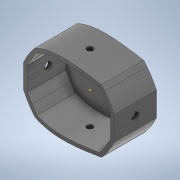
# Autodesk Inventor part: CameraHolder2
Saved by Autodesk Inventor 2021.1 (Build 251245010, 245A)
## iProperties
Created: 2023-07-02
Part Number: CameraHolder2
Material: ABS Plastic
Document SubType Name: Modeling
Designer: Drake
Density: 1.06 g/cm^3
Appearance: Smooth - White
Author: Drake
Autodesk Inventor part; units mm, degrees
ref_plane "XY Plane" through (0, 0, 0) normal (0, 0, 1) x (1, 0, 0)
sketch "Sketch1" plane through (0, 0, 0) normal (0, 0, 1) x (1, 0, 0)
  circle A0 centre (0, 0) radius 75
  line L0 (-56.086285, 49.792857) -> (-26.079044, 63.659157) construction
  line L1 (-26.079044, 63.659157) -> (7.211359, 60.092328) construction
  line L2 (7.211359, 60.092328) -> (53.805209, 52.249397) construction
  spline S0 degree 3 poles (-56.086285, 49.792857) (-26.079044, 63.659157) (7.211359, 60.092328) (53.805209, 52.249397) knots 1 1 1 1 2 2 2 2
  line L3 (-75, 0) -> (75, 0)
  line L4 (-56.086285, -49.792857) -> (-26.079044, -63.659157) construction
  line L5 (-26.079044, -63.659157) -> (7.211359, -60.092328) construction
  line L6 (7.211359, -60.092328) -> (53.805209, -52.249397) construction
  spline S1 degree 3 poles (-56.086285, -49.792857) (-26.079044, -63.659157) (7.211359, -60.092328) (53.805209, -52.249397) knots 1 1 1 1 2 2 2 2
  line L7 (0, 0) -> (0, 49.151954)
  line L8 (-75, 0) -> (-75, 20)
  line L9 (-75, 20) -> (-75, -20)
  line L10 (0, 49.151954) -> (0, -37.368697)
  line L11 (75, 20) -> (75, -20)
  arc A1 (-56.086285, 49.792857) -> (-75, 20) centre (35.126867, -29.012979) ccw
  line L12 (0, 49.151954) -> (0, 75)
  line L13 (0, 75) -> (0, -75.710243)
  line L14 (-75, 0) -> (75, 0)
  arc A2 (75, 20) -> (56.086285, 49.792857) centre (-35.126867, -29.012979) ccw
  line L15 (-115.860838, 0) -> (95.477913, 0)
  line L16 (-56.086285, -49.792857) -> (-26.079044, -63.659157) construction
  line L17 (-26.079044, -63.659157) -> (7.211359, -60.092328) construction
  line L18 (7.211359, -60.092328) -> (53.805209, -52.249397) construction
  spline S2 degree 3 poles (-56.086285, -49.792857) (-26.079044, -63.659157) (7.211359, -60.092328) (53.805209, -52.249397) knots 1 1 1 1 2 2 2 2
  arc A3 (-75, -20) -> (-56.086285, -49.792857) centre (35.126867, 29.012979) ccw
  arc A4 (56.086285, -49.792857) -> (75, -20) centre (-35.126867, 29.012979) ccw
  point P0 (0, 4.953623)
  point P1 (0, 5)
  point P2 (0.109556, -4.9988)
  point P3 (0.109556, 4.9988)
  point P4 (-59.492302, -45.669092)
  point P5 (-59.492302, 45.669092)
  point P6 (59.492302, -45.669092)
  point P7 (59.492302, 45.669092)
  dimension "d11" = 49.15195
  dimension "motorlw" = 20
  dimension "d19" = 40
  constraints: 20 end point, 13 point on circle, 11 symmetric about line, 5 centre point, 4 point on line, 3 vertical, 1 coincident, 1 collinear, 1 horizontal, 1 tangent, 12 other
  measures "d11" distance of L7.start L7.end
  measures "motorlw" distance of L3.start L8.end
  measures "d19" distance of L8.end L9.end
sketch "Sketch2" plane through (0, 0, 0) normal (1, 0, 0) x (0, 1, 0)
  point P0 (0, 0)
extrude "Extrusion1" add sketch "Sketch1" against normal mid plane 70 contours A2 A0 L3 L7 L12 S0 | A0 A2 | A2 L11 A0 | L12 L7 L3 A0 A1 S0 | L11 A4 A0 | A0 A4 S1 L13 L10 L3 | A1 A0 | A0 A4 | L10 L13 S1 A3 A0 L3 | A0 L8 A1 | A0 A3 L9 | A3 A0
sketch "Sketch3" plane through (0, 0, 35) normal (0, 0, 1) x (1, 0, 0)
  spline S0 degree 3 poles (53.805209, 52.249397) (7.211359, 60.092328) (-26.079044, 63.659157) (-56.086285, 49.792857) knots 0 0 0 0 1 1 1 1
  arc A0 (-56.086285, 49.792857) -> (-56.086285, -49.792857) centre (0, 0) ccw
  arc A1 (53.805209, -52.249397) -> (53.805209, 52.249397) centre (0, 0) ccw
  spline S1 degree 3 poles (-56.086285, -49.792857) (-26.079044, -63.659157) (7.211359, -60.092328) (53.805209, -52.249397) knots 0 0 0 0 1 1 1 1
  arc A2 (50.826915, -46.665026) -> (50.826915, 46.665026) centre (0, 0) ccw
  arc A3 (-52.420696, 44.867256) -> (-52.420696, -44.867256) centre (0, 0) ccw
  arc A4 (-59.492302, 45.669092) -> (-75, 20) centre (35.126867, -29.012979) ccw
  line L0 (-75, 20) -> (-75, -20)
  arc A5 (-75, -20) -> (-59.492302, -45.669092) centre (35.126867, 29.012979) ccw
  arc A6 (59.492302, -45.669092) -> (75, -20) centre (-35.126867, 29.012979) ccw
  line L1 (75, -20) -> (75, 20)
  arc A7 (75, 20) -> (59.492302, 45.669092) centre (-35.126867, -29.012979) ccw
  arc A8 (69, 18.708077) -> (54.782588, 41.951756) centre (-35.126867, -29.012979) ccw
  line L2 (69, 18.708077) -> (69, -18.708077)
  arc A9 (54.782588, -41.951756) -> (69, -18.708077) centre (-35.126867, 29.012979) ccw
  arc A10 (-54.782588, 41.951756) -> (-69, 18.708077) centre (35.126867, -29.012979) ccw
  line L3 (-69, 18.708077) -> (-69, -18.708077)
  arc A11 (-69, -18.708077) -> (-54.782588, -41.951756) centre (35.126867, 29.012979) ccw
  line L4 (-69, 18.708077) -> (-52.420696, 44.867256)
  line L5 (-69, 18.708077) -> (-69, -18.708077)
  line L6 (-75, -20) -> (-75, 20)
  line L7 (50.826915, -46.665026) -> (69, -18.708077)
  line L8 (69, 18.708077) -> (50.826915, 46.665026)
  line L9 (-69, 18.708077) -> (-69, -18.708077)
  line L10 (-52.420696, -44.867256) -> (-36.895618, -50.128134)
  line L11 (-69, 0) -> (-68.398162, -20)
  line L12 (-60.766679, -32.686552) -> (-68.398162, -20)
  spline S2 degree 5 poles (-52.420671, 44.8672) (-47.019003, 47.270944) (-41.416917, 49.227592) (-35.660804, 50.693332) (-22.969469, 52.923431) (-10.081677, 53.395428) (-3.126582, 53.253873) (11.898151, 52.342936) (26.833492, 50.455881) (34.844576, 49.277842) (42.840453, 47.998688) (50.826911, 46.664999) knots 0 0 0 0 0 0 0.28211477 0.28211477 0.28211477 0.61364676 0.61364676 0.61364676 1 1 1 1 1 1
  spline S3 degree 5 poles (50.826911, -46.664999) (42.840453, -47.998688) (34.844576, -49.277842) (26.833492, -50.455881) (11.898151, -52.342936) (-3.126582, -53.253873) (-10.081677, -53.395428) (-22.969469, -52.923431) (-35.660804, -50.693332) (-41.416917, -49.227592) (-47.019003, -47.270944) (-52.420671, -44.8672) knots 0 0 0 0 0 0 0.38635324 0.38635324 0.38635324 0.71788523 0.71788523 0.71788523 1 1 1 1 1 1
  point P0 (63.279421, 27.508451)
  point P1 (69, 0)
  point P2 (63.279421, -27.508451)
  point P3 (-62.950405, 28.253257)
  point P4 (-69, 0)
  point P5 (-68.875151, -4.148928)
  dimension "d4" = 6
  dimension "d20" = 6
  dimension "d21" = 6
  constraints: 20 end point, 14 point on circle, 6 centre point, 3 concentric, 1 collinear, 1 midpoint, 1 parallel, 13 other
  measures "d20" radial gap between concentric circles of A7 A8
  measures "d21" radial gap between concentric circles of A4 A10
extrude "Extrusion2" cut sketch "Sketch3" against normal blind 64 contours L7 A2 | S3 L10 A3 L11 L4 S2 L8 A2 L7 | A2 L2 L7 | S3 L10 | A2 L8 L2 | L8 A2 | L12 L11 A3 | L4 A3 | A3 L11 | A3 L3 L4
ref_plane "Work Plane1" through (60, 0, 0) normal (1, 0, 0) x (0, 1, 0)
sketch "Sketch4" plane through (60, 0, 0) normal (1, 0, 0) x (0, 1, 0)
  arc A0 (5.8125, 1.488235) -> (5.8125, -1.488235) centre (0, 0) ccw
  arc A1 (5.8125, -1.488235) -> (5.8125, 1.488235) centre (6, 0) ccw
  dimension "motorcrescenttop" = 12
  dimension "crescent" = 3
  constraints: 5 point on circle, 2 centre point, 1 coincident
  measures "motorcrescenttop" diameter of A0
  measures "crescent" diameter of A1
extrude "Extrusion3" cut sketch "Sketch4" against normal mid plane 300
ref_plane "Work Plane2" through (0, 49.152, 0) normal (0, 1, 0) x (-1, 0, 0)
sketch "Sketch5" plane through (0, 49.152, 0) normal (0, 1, 0) x (-1, 0, 0)
  circle A0 centre (0, 0) radius 5
  dimension "d13" = 10
  constraints: 1 centre point, 1 coincident
  measures "d13" diameter of A0
mirror "Mirror1" about plane through (0, 0, 0) normal (0, 0, 1) of "Extrusion3"
ref_plane "Work Plane3" through (70, 0, 0) normal (1, 0, 0) x (0, 1, 0)
extrude "Extrusion4" cut sketch "Sketch5" against normal through all both and the other way through all
equation "\"d2\" = d1"
equation "\"d1\" = 70"
body "Solid1"
